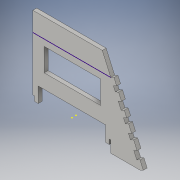
# Autodesk Inventor part: mcdave_rail2
Saved by Autodesk Inventor 2016 (Build 200138000, 138)
## iProperties
Created: 2017-11-29
Part Number: mcdave_rail2
Material: Generic
Document SubType Name: Modeling
Designer: student
Density: 1 g/cm^3
Appearance: Default
Author: student
Autodesk Inventor part; units mm, degrees
ref_plane "YZ Plane" through (0, 0, 0) normal (1, 0, 0) x (0, 1, 0)
ref_plane "XZ Plane" through (0, 0, 0) normal (0, 1, 0) x (-1, 0, 0)
ref_plane "XY Plane" through (0, 0, 0) normal (0, 0, 1) x (1, 0, 0)
sketch "Sketch1" plane through (0, 0, 0) normal (0, 0, 1) x (1, 0, 0)
  line L0 (-27.9942, -0.0006) -> (-27.9942, -3.8862)
  line L1 (-27.9942, -3.8862) -> (-31.22, -3.8862)
  line L2 (27.7334, 0) -> (27.7334, -3.8862)
  line L3 (-31.22, -3.8862) -> (-31.22, 45.0041)
  line L4 (27.7334, -3.8862) -> (30.9592, -3.8862)
  line L5 (30.9592, -3.8862) -> (30.9592, 45.0041)
  line L6 (30.9592, 45.0041) -> (-31.22, 45.0041)
  line L7 (27.7334, -3.8862) -> (27.7334, 0)
  line L8 (27.7334, 0) -> (27.7334, 6.9041)
  line L9 (27.7334, 6.9041) -> (-27.9942, 6.9041)
  line L10 (-27.9942, 6.9041) -> (-27.9942, -0.0006)
  line L11 (30.9592, 6.9041) -> (-31.22, 6.9041)
  point P0 (0, 0)
  point P1 (27.7334, 4.1367)
  dimension "d3" = 3.2258
  dimension "d4" = 55.7276
  dimension "d5" = 3.2258
  dimension "d33" = 38.1
  constraints: 24 end point, 4 point on line, 4 vertical, 3 perpendicular, 2 horizontal, 1 collinear
  measures "d3" distance of L0.end L1.end
  measures "d4" distance of L0.start L2.start
  measures "d5" distance of L2.end L4.end
  measures "d33" distance between parallel lines of L9 L6
extrude "Extrusion1" add sketch "Sketch1" along normal blind 3.2258
sketch "Sketch2" plane through (30.9592, -3.8862, 0) normal (1, 0, 0) x (0, 0, -1)
  point P0 (0, 3.8862)
sketch "Sketch4" plane through (0, 0, 0) normal (0, 0, -1) x (-1, 0, 0)
  point P0 (0, 0)
sketch "Sketch5" plane through (0, 0, 0) normal (0, 0, -1) x (-1, 0, 0)
  line L0 (-30.9592, -3.8862) -> (-30.9592, 45.0041) projected
  line L1 (-30.9592, 0) -> (-30.9592, -1.27)
  line L2 (-30.9592, 0) -> (-32.2292, 0)
  line L3 (-32.2292, 0) -> (-32.2292, 45.0041)
  line L4 (-32.2292, 45.0041) -> (-30.9592, 45.0041)
  line L5 (-30.9592, 45.0041) -> (31.22, 45.0041) projected
  line L6 (0.1304, 45.0041) -> (0.1304, 20.6375)
  line L7 (31.22, 0) -> (32.49, 0)
  line L8 (32.49, 0) -> (32.49, 45.0041)
  line L9 (32.49, 45.0041) -> (31.22, 45.0041)
  line L10 (31.22, 45.0041) -> (31.22, -3.8862) projected
  point P0 (0, 0)
  point P1 (-21.0964, 42.2367)
  point P2 (21.0964, 42.2367)
  point P3 (31.22, 0)
  dimension "d14" = 1.27
  dimension "d15" = 1.27
  constraints: 16 end point, 4 point on line, 4 symmetric about line, 2 vertical, 1 horizontal, 1 perpendicular, 2 other
  measures "d14" distance of L1.start L1.end
  measures "d15" distance of L1.start L2.end
extrude "Extrusion3" add sketch "Sketch5" against normal blind 3.2258
sketch "Sketch10" plane through (0, 0, 0) normal (0, 0, -1) x (-1, 0, 0)
  point P0 (0, 0)
sketch "Sketch11" plane through (0, 0, 0) normal (0, 0, -1) x (-1, 0, 0)
  point P0 (0, 0)
sketch "Sketch13" plane through (0, 0, 0) normal (0, 0, -1) x (-1, 0, 0)
  line L0 (-32.2292, 45.0041) -> (-32.2292, 0) projected
  line L1 (-32.2292, 45.0041) -> (27.4604, 45.0041) construction
  line L2 (-56.5071, -9.525) -> (-32.8958, -9.525)
  line L3 (-32.2292, 0) -> (-30.9592, 0) projected
  line L4 (-32.2292, 0) -> (-32.2292, -9.525)
  line L5 (-32.2292, -9.525) -> (-32.8958, -9.525)
  line L6 (-34.925, 46.2044) -> (-32.2292, 45.0041)
  line L7 (-59.2029, -8.3247) -> (-56.5071, -9.525)
  line L8 (-56.5071, -2.2699) -> (-53.8113, -3.4701)
  line L9 (-53.8113, 3.175) -> (-51.3422, 2.0757)
  line L10 (-37.1197, 41.275) -> (-34.4239, 40.0747)
  line L11 (-36.0254, 36.4778) -> (-38.7212, 37.678)
  line L12 (-38.4353, 31.0649) -> (-41.1312, 32.2651)
  line L13 (-34.925, 46.2044) -> (-37.1197, 41.275)
  line L14 (-38.7212, 37.678) -> (-41.1312, 32.2651)
  line L15 (-56.5071, -2.2699) -> (-59.2029, -8.3247)
  line L16 (-51.2557, 9.525) -> (-48.5599, 8.3247)
  line L17 (-59.2029, -8.3247) -> (-56.5071, -2.2699)
  line L18 (-53.8113, 3.175) -> (-54.038, 3.2759)
  line L19 (-56.5071, -2.2699) -> (-59.2029, -8.3247)
  line L20 (-49.5406, 13.3771) -> (-46.8448, 12.1769)
  line L21 (-47.0149, 19.05) -> (-44.3682, 17.7396)
  line L22 (-45.478, 22.5021) -> (-42.7821, 21.3018)
  line L23 (-43.4768, 26.9966) -> (-40.781, 25.7964)
  line L24 (-34.925, 46.2044) -> (-37.1197, 41.275)
  line L25 (-38.7212, 37.678) -> (-41.1312, 32.2651)
  line L26 (-49.5406, 13.3771) -> (-47.0149, 19.05)
  line L27 (-45.478, 22.5021) -> (-43.4768, 26.9966)
  line L28 (-47.0149, 19.05) -> (-49.5406, 13.3771)
  line L29 (-51.2557, 9.525) -> (-54.038, 3.2759)
  line L30 (-51.3422, 2.0757) -> (-53.8113, -3.4701)
  line L31 (-46.8448, 12.1769) -> (-48.5599, 8.3247)
  line L32 (-42.7821, 21.3018) -> (-44.3682, 17.7396)
  line L33 (-34.4239, 40.0747) -> (-36.0254, 36.4778)
  line L34 (-38.4353, 31.0649) -> (-40.781, 25.7964)
  point P0 (0, 0)
  constraints: 66 end point, 50 perpendicular, 8 collinear, 1 horizontal, 1 vertical
extrude "Extrusion8" add sketch "Sketch13" against normal blind 3.2258
sketch "Sketch14" plane through (0, 0, 3.2258) normal (0, 0, 1) x (1, 0, 0)
  line L0 (-32.49, 45.0041) -> (32.2292, 45.0041) projected
  line L1 (-23.0867, 39.6875) -> (-23.0867, 31.75)
  line L2 (23.8125, 31.75) -> (23.8125, 39.6875)
  line L3 (-23.0867, 31.75) -> (-23.0867, 28.575)
  line L4 (23.8125, 28.575) -> (23.8125, 31.75)
  line L5 (-23.0867, 39.6875) -> (23.8125, 39.6875)
  line L6 (-23.0867, 28.575) -> (-23.0867, 20.6375)
  line L7 (-23.0867, 20.6375) -> (23.8125, 20.6375)
  line L8 (23.8125, 20.6375) -> (23.8125, 28.575)
  point P0 (0, 0)
  point P1 (-27.9942, 45.0041)
  point P2 (27.7334, 45.0041)
  constraints: 16 end point, 3 perpendicular, 3 vertical
extrude "Extrusion9" cut sketch "Sketch14" against normal through all
sketch "Sketch15" plane through (0, 0, 0) normal (0, 0, -1) x (-1, 0, 0)
  line L0 (27.9942, 6.9041) -> (-27.7334, 6.9041) projected
  line L1 (-27.7334, 6.9041) -> (-27.7334, 8.7347)
  line L2 (-27.7334, 8.7347) -> (27.9942, 8.7347)
  line L3 (27.9942, 8.7347) -> (27.9942, 6.9041)
  point P0 (0, 0)
  constraints: 6 end point, 2 perpendicular, 1 vertical
extrude "Extrusion10" cut sketch "Sketch15" against normal through all
sketch "Sketch16" plane through (0, 0, 3.2258) normal (0, 0, 1) x (1, 0, 0)
  line L0 (37.1197, 41.275) -> (34.4239, 40.0747) projected
  line L1 (34.4239, 40.0747) -> (29.6487, 50.8)
  line L2 (34.4239, 40.0747) -> (46.1641, 40.0747) construction
  line L3 (-32.49, 45.0041) -> (-32.49, 0) projected
  line L4 (-32.49, 45.0041) -> (-32.49, 60.9185)
  line L5 (-32.49, 60.9185) -> (25.1436, 60.9185)
  line L6 (25.1436, 60.9185) -> (29.6487, 50.8)
  line L7 (-32.49, 45.0041) -> (32.2292, 45.0041) projected
  line L8 (-32.49, 45.0041) -> (32.2292, 45.0041)
  line L9 (-31.22, 48.8903) -> (-31.22, 45.0041) projected
  line L10 (-31.22, 45.0041) -> (-31.22, 48.8903)
  line L11 (-31.22, 48.8903) -> (-28.575, 48.8903)
  line L12 (-31.22, 48.8903) -> (-27.9942, 48.8903) projected
  line L13 (-27.9942, 48.8903) -> (-27.9942, 45.0041) projected
  line L14 (-27.9942, 48.8903) -> (-27.9942, 45.0041)
  line L15 (-32.49, 45.0041) -> (32.2292, 45.0041) projected
  line L16 (27.7334, 45.0041) -> (27.7334, 48.8903) projected
  line L17 (27.7334, 45.0041) -> (27.7334, 48.8903)
  line L18 (27.7334, 48.8903) -> (30.9592, 48.8903) projected
  line L19 (27.7334, 48.8903) -> (30.9592, 48.8903)
  line L20 (-29.187, 48.8903) -> (-27.9942, 48.8903)
  line L21 (32.2292, 45.0041) -> (34.925, 46.2044) projected
  line L22 (-32.49, 45.0041) -> (32.2292, 45.0041)
  line L23 (25.1436, 60.9185) -> (32.2292, 45.0041)
  point P0 (0, 0)
  point P1 (30.9592, 45.0041)
  dimension "d47" = 114
  constraints: 28 end point, 4 collinear, 4 perpendicular, 2 horizontal, 2 vertical, 1 equal length, 1 point on line
  measures "d47" angle of L2 L1
sketch "Sketch17" plane through (0, 0, 3.2258) normal (0, 0, 1) x (1, 0, 0)
  line L0 (-32.49, 45.0041) -> (32.2292, 45.0041) projected
  line L1 (-32.49, 45.0041) -> (32.2292, 45.0041)
  point P0 (0, 0)
  constraints: 2 end point, 1 collinear
extrude "Extrusion11" add sketch "Sketch16" against normal blind 3.2258
body "Solid1"
